Autodesk Inventor part; units mm, degrees
(part 2 of 2)
sketch "스케치25" plane through (0, 0, 3) normal (0, 0, 1) x (1, 0, 0)
  arc A0 (-11.265, 4.4922) -> (-11.1472, 2.4957) centre (-11.2061, 3.4939) ccw projected
  arc A1 (-11.1472, -2.4957) -> (-11.1472, 2.4957) centre (-11, 0) ccw projected
  arc A2 (-11.1472, -2.4957) -> (-12.1608, -3.7916) centre (-11.2061, -3.4939) ccw projected
  arc A3 (-12.1608, -3.7916) -> (-11.28, -5.9179) centre (0, 0) ccw projected
  arc A4 (-11.28, -5.9179) -> (-9.647, -6.1176) centre (-10.3945, -5.4533) ccw projected
  arc A5 (-7.0945, -10.1829) -> (-9.647, -6.1176) centre (-7.7782, -7.7782) ccw projected
  arc A6 (-7.0945, -10.1829) -> (-7.6646, -11.6816) centre (-6.821, -11.1447) ccw projected
  line L0 (-4.7245, -16.3015) -> (-7.6646, -11.6816) projected
  arc A7 (-3.9745, -19.5493) -> (-4.7245, -16.3015) centre (-8.9427, -18.986) ccw projected
  arc A8 (-3.9745, -19.5493) -> (3.9745, -19.5493) centre (0, -20) ccw projected
  arc A9 (4.7245, -16.3015) -> (3.9745, -19.5493) centre (8.9427, -18.986) ccw projected
  line L1 (7.6646, -11.6816) -> (4.7245, -16.3015) projected
  arc A10 (7.6646, -11.6816) -> (7.0945, -10.1829) centre (6.821, -11.1447) ccw projected
  arc A11 (9.647, -6.1176) -> (7.0945, -10.1829) centre (7.7782, -7.7782) ccw projected
  arc A12 (9.647, -6.1176) -> (11.28, -5.9179) centre (10.3945, -5.4533) ccw projected
  arc A13 (11.28, -5.9179) -> (12.1608, -3.7916) centre (0, 0) ccw projected
  arc A14 (12.1608, -3.7916) -> (11.1472, -2.4957) centre (11.2061, -3.4939) ccw projected
  arc A15 (11.1472, 2.4957) -> (11.1472, -2.4957) centre (11, 0) ccw projected
  arc A16 (11.1472, 2.4957) -> (11.265, 4.4922) centre (11.2061, 3.4939) ccw projected
  arc A17 (11.265, 4.4922) -> (6.5, 0) centre (11, 0) ccw projected
  arc A18 (-6.5, 0) -> (6.5, 0) centre (0, 0) ccw projected
  arc A19 (-6.5, 0) -> (-11.265, 4.4922) centre (-11, 0) ccw projected
  circle A20 centre (0, -20) radius 2.05 projected
  line L2 (-2.4969, -11.125) -> (-2.2662, -15.7322) projected
  arc A21 (2.4969, -11.125) -> (-2.4969, -11.125) centre (0, -11) ccw projected
  line L3 (2.2662, -15.7322) -> (2.4969, -11.125) projected
  arc A22 (0.9858, -16.6417) -> (2.2662, -15.7322) centre (1.2675, -15.6822) ccw projected
  arc A23 (0.9858, -16.6417) -> (-0.9858, -16.6417) centre (0, -20) ccw projected
  arc A24 (-2.2662, -15.7322) -> (-0.9858, -16.6417) centre (-1.2675, -15.6822) ccw projected
extrude "돌출24" add sketch "스케치25" against normal up to surface (3 mm away) contours A21 L3 A22 A23 A24 L2
